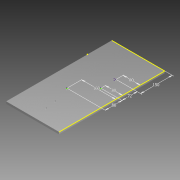
# Autodesk Inventor part: Wand rechts
Saved by Autodesk Inventor 2013 (Build 170138000, 138)
## iProperties
Created: 2012-10-20
Part Number: Wand rechts
Material: Acryl, farblos
Document SubType Name: Modeling
Designer: fivef
Density: 1.19 g/cm^3
Mass: 1782.71 g
Surface Area: 3177.15 cm^2
Volume: 1498.08 cm^3
Author: fivef
Autodesk Inventor part; units mm, degrees
ref_plane "YZ Plane" through (0, 0, 0) normal (1, 0, 0) x (0, 1, 0)
ref_plane "XZ Plane" through (0, 0, 0) normal (0, 1, 0) x (-1, 0, 0)
ref_plane "XY Plane" through (0, 0, 0) normal (0, 0, 1) x (1, 0, 0)
sketch "Skizze1" plane through (0, 0, 0) normal (0, 0, 1) x (1, 0, 0)
  line L0 (0, 115.5102) -> (250, 115.5102)
  line L1 (250, 115.5102) -> (250, -384.4898)
  line L2 (250, -384.4898) -> (0, -384.4898)
  line L3 (0, -384.4898) -> (0, 115.5102)
  point P0 (0, 0)
  point P1 (190, -104.4898)
  dimension "d0" = 250
  dimension "d2" = 500
  dimension "d3" = 60
  dimension "d4" = 220
  constraints: 8 end point, 2 parallel, 1 horizontal, 1 perpendicular
  measures "d0" distance of L1.end L2.end
  measures "d2" distance of L0.end L1.end
  measures "d3" distance from line of L1 point (190, -104.49)
  measures "d4" distance from line of L0 point (190, -104.49)
extrude "Extrusion1" add sketch "Skizze1" along normal blind 10
sketch "Skizze3" plane through (0, 0, 10) normal (0, 0, 1) x (1, 0, 0)
  circle A0 centre (90, -186.4898) radius 3
  circle A1 centre (170, -106.4898) radius 3
  line L0 (250, 115.5102) -> (0, 115.5102) projected
  line L1 (250, -384.4898) -> (250, 115.5102) projected
  point P0 (0, 0)
  point P1 (170, -34.4898)
  dimension "d30" = 80
  dimension "d36" = 150
  dimension "d69" = 160
  dimension "d70" = 72
  dimension "d72" = 80
  dimension "d73" = 80
  constraints: 2 centre point
  measures "d30" distance from line of L1 point (170, -34.49)
  measures "d36" distance from line of L0 point (170, -34.49)
  measures "d69" distance from line of L1 A0.centre
  measures "d70" distance of point (170, -34.49) A1.centre
  measures "d72" distance from line of L1 A1.centre
  measures "d73" horizontal distance of A0.centre A1.centre
hole "Bohrung3" at (90, -186.4898, 10) at (170, -106.4898, 10) at (170, -34.4898, 10) direction (0, 0, -1) diameter 4.3 end through all
sketch "Skizze5" plane through (0, 0, 10) normal (0, 0, 1) x (1, 0, 0)
  point P0 (0, 0)
  point P1 (115, -266.4898)
  point P2 (122, -316.4898)
  point P3 (90, -186.4898)
  dimension "d74" = 50
  dimension "d75" = 25
  dimension "d76" = 7
  dimension "d77" = 80
  measures "d74" vertical distance of point (115, -266.49) point (122, -316.49)
  measures "d75" horizontal distance of point (90, -186.49) point (115, -266.49)
  measures "d76" horizontal distance of point (115, -266.49) point (122, -316.49)
  measures "d77" vertical distance of point (90, -186.49) point (115, -266.49)
hole "Bohrung4" at (115, -266.4898, 10) at (122, -316.4898, 10) direction (0, 0, -1) diameter 4.3 end through all
